Autodesk Fusion 360 part; units mm, degrees
(part 2 of 4)
sketch "top profile" plane through (0, 0, 1.6) normal (0, 0, 1) x (-1, 0, 0)
  circle A0 centre (-116.1773, 3.3688) radius 1.55
  line L0 (-280.938, -16.8245) -> (-266.937, -16.8245)
  line L1 (-266.937, -16.8245) -> (-266.937, -30.824)
  line L2 (-266.937, -30.824) -> (-280.938, -30.824)
  line L3 (-280.938, -30.824) -> (-280.938, -16.8245)
  line L4 (-197.772, -48.7839) -> (-183.986, -46.3532)
  line L5 (-183.986, -46.3532) -> (-181.555, -60.1405)
  line L6 (-181.555, -60.1405) -> (-195.341, -62.5711)
  line L7 (-195.341, -62.5711) -> (-197.772, -48.7839)
  line L8 (-176.582, -59.2624) -> (-179.013, -45.4752)
  line L9 (-179.013, -45.4752) -> (-165.224, -43.0445)
  line L10 (-165.224, -43.0445) -> (-162.793, -56.8318)
  line L11 (-162.793, -56.8318) -> (-176.582, -59.2624)
  line L12 (-45.4822, -49.874) -> (-59.4815, -49.874)
  line L13 (-59.4815, -49.874) -> (-59.4815, -35.8743)
  line L14 (-59.4815, -35.8743) -> (-45.4822, -35.8743)
  line L15 (-45.4822, -35.8743) -> (-45.4822, -49.874)
  line L16 (-176.444, -20.5521) -> (-190.233, -22.9829)
  line L17 (-190.233, -22.9829) -> (-192.664, -9.1956)
  line L18 (-192.664, -9.1957) -> (-178.876, -6.7634)
  line L19 (-178.876, -6.7634) -> (-176.444, -20.5521)
  line L20 (-281.226, -49.874) -> (-295.225, -49.874)
  line L21 (-295.225, -49.874) -> (-295.225, -35.8743)
  line L22 (-295.225, -35.8743) -> (-281.226, -35.8743)
  line L23 (-281.226, -35.8743) -> (-281.226, -49.874)
  line L24 (-109.921, -22.1561) -> (-123.708, -19.7253)
  line L25 (-123.708, -19.7253) -> (-121.277, -5.9366)
  line L26 (-121.277, -5.9366) -> (-107.49, -8.3688)
  line L27 (-107.49, -8.3688) -> (-109.921, -22.1561)
  line L28 (-349.994, -68.924) -> (-349.994, -54.9243)
  line L29 (-349.994, -54.9243) -> (-335.995, -54.9243)
  line L30 (-335.995, -54.9243) -> (-335.995, -68.924)
  line L31 (-335.995, -68.924) -> (-349.994, -68.924)
  line L32 (-257.125, -16.8245) -> (-243.126, -16.8245)
  line L33 (-243.126, -16.8245) -> (-243.126, -30.824)
  line L34 (-243.126, -30.824) -> (-257.125, -30.824)
  line L35 (-257.125, -30.824) -> (-257.125, -16.8245)
  line L36 (-12.1447, -73.9743) -> (-12.1447, -87.974)
  line L37 (-12.1447, -87.974) -> (-26.1441, -87.974)
  line L38 (-26.1441, -87.974) -> (-26.1441, -73.9743)
  line L39 (-26.1441, -73.9743) -> (-12.1447, -73.9743)
  line L40 (-193.416, -100.919) -> (-195.847, -87.1319)
  line L41 (-195.847, -87.1319) -> (-182.059, -84.7012)
  line L42 (-182.059, -84.7012) -> (-179.629, -98.4885)
  line L43 (-179.629, -98.4885) -> (-193.416, -100.919)
  line L44 (-177.086, -83.8232) -> (-163.299, -81.3925)
  line L45 (-163.299, -81.3925) -> (-160.868, -95.1812)
  line L46 (-160.868, -95.1812) -> (-174.655, -97.6119)
  line L47 (-174.655, -97.6119) -> (-177.086, -83.8232)
  line L48 (-189.775, -66.7177) -> (-175.988, -64.2867)
  line L49 (-175.988, -64.2867) -> (-173.557, -78.0743)
  line L50 (-173.557, -78.0743) -> (-187.343, -80.5049)
  line L51 (-187.343, -80.5049) -> (-189.775, -66.7177)
  line L52 (-200.82, -88.0085) -> (-198.389, -101.797)
  line L53 (-198.389, -101.797) -> (-212.176, -104.228)
  line L54 (-212.176, -104.228) -> (-214.607, -90.4392)
  line L55 (-214.607, -90.4392) -> (-200.82, -88.0085)
  line L56 (-117.5, -78.8515) -> (-131.287, -76.4205)
  line L57 (-131.287, -76.4205) -> (-128.856, -62.6332)
  line L58 (-128.856, -62.6332) -> (-115.069, -65.0642)
  line L59 (-115.069, -65.0642) -> (-117.5, -78.8515)
  line L60 (-111.428, -99.2657) -> (-125.214, -96.8347)
  line L61 (-125.214, -96.8347) -> (-122.783, -83.0474)
  line L62 (-122.783, -83.0474) -> (-108.996, -85.4784)
  line L63 (-108.996, -85.4784) -> (-111.428, -99.2657)
  circle A1 centre (-309.1199, -118.074) radius 1.55
  line L64 (-12.1447, -93.0243) -> (-12.1447, -107.024)
  line L65 (-12.1447, -107.024) -> (-26.1441, -107.024)
  line L66 (-26.1441, -107.024) -> (-26.1441, -93.0243)
  line L67 (-26.1441, -93.0243) -> (-12.1447, -93.0243)
  line L68 (-143.976, -93.5274) -> (-141.544, -79.7387)
  line L69 (-141.544, -79.7387) -> (-127.758, -82.1697)
  line L70 (-127.758, -82.1697) -> (-130.189, -95.9584)
  line L71 (-130.189, -95.9584) -> (-143.976, -93.5274)
  line L72 (-194.747, -67.5954) -> (-192.316, -81.3816)
  line L73 (-192.316, -81.3816) -> (-206.105, -83.8122)
  line L74 (-206.105, -83.8122) -> (-208.536, -70.0264)
  line L75 (-208.536, -70.0264) -> (-194.747, -67.5954)
  line L76 (-49.9565, -87.974) -> (-49.9565, -73.9743)
  line L77 (-49.9565, -73.9743) -> (-35.9572, -73.9743)
  line L78 (-35.9572, -73.9743) -> (-35.9572, -87.974)
  line L79 (-35.9572, -87.974) -> (-49.9565, -87.974)
  arc A2 (-176.1339, -7.7732) -> (-176.9451, -8.9317) centre (-175.9603, -8.758) ccw
  line L80 (-176.1339, -7.7732) -> (-170.6459, -6.8059)
  arc A3 (-169.4875, -7.6172) -> (-170.6459, -6.8059) centre (-170.4724, -7.7907) ccw
  line L81 (-169.4875, -7.6172) -> (-167.4915, -18.9424)
  arc A4 (-168.3027, -20.1008) -> (-167.4915, -18.9424) centre (-168.4764, -19.116) ccw
  line L82 (-168.3027, -20.1008) -> (-173.7893, -21.0686)
  arc A5 (-174.9478, -20.2574) -> (-173.7893, -21.0686) centre (-173.963, -20.0838) ccw
  line L83 (-174.9478, -20.2574) -> (-176.9451, -8.9317)
  line L84 (-255.032, -49.874) -> (-269.032, -49.874)
  line L85 (-269.032, -49.874) -> (-269.032, -35.8743)
  line L86 (-269.032, -35.8743) -> (-255.032, -35.8743)
  line L87 (-255.032, -35.8743) -> (-255.032, -49.874)
  line L88 (-98.9566, -12.3811) -> (-100.9548, -23.7064)
  arc A6 (-102.1133, -24.5174) -> (-100.9548, -23.7064) centre (-101.9395, -23.5327) ccw
  line L89 (-102.1133, -24.5174) -> (-107.6038, -23.5487)
  arc A7 (-108.4148, -22.3903) -> (-107.6038, -23.5487) centre (-107.43, -22.564) ccw
  line L90 (-108.4148, -22.3903) -> (-106.4177, -11.0651)
  arc A8 (-105.2592, -10.254) -> (-106.4177, -11.0651) centre (-105.4329, -11.2388) ccw
  line L91 (-105.2592, -10.254) -> (-99.7677, -11.2225)
  arc A9 (-98.9566, -12.3811) -> (-99.7677, -11.2225) centre (-99.9414, -12.2073) ccw
  line L92 (-132.669, -56.8318) -> (-130.238, -43.0445)
  line L93 (-130.238, -43.0445) -> (-116.451, -45.4752)
  line L94 (-116.451, -45.4752) -> (-118.882, -59.2624)
  line L95 (-118.882, -59.2624) -> (-132.669, -56.8318)
  line L96 (-249.982, -49.874) -> (-249.982, -35.8743)
  line L97 (-249.982, -35.8743) -> (-235.982, -35.8743)
  line L98 (-235.982, -35.8743) -> (-235.982, -49.874)
  line L99 (-235.982, -49.874) -> (-249.982, -49.874)
  line L100 (-106.193, -42.1569) -> (-119.98, -39.726)
  line L101 (-119.98, -39.726) -> (-117.549, -25.9388)
  line L102 (-117.549, -25.9388) -> (-103.762, -28.3697)
  line L103 (-103.762, -28.3697) -> (-106.193, -42.1569)
  line L104 (-28.5254, -35.8743) -> (-14.5259, -35.8743)
  line L105 (-14.5259, -35.8743) -> (-14.5259, -49.874)
  line L106 (-14.5259, -49.874) -> (-28.5254, -49.874)
  line L107 (-28.5254, -49.874) -> (-28.5254, -35.8743)
  line L108 (-136.31, -22.6315) -> (-122.524, -25.0624)
  line L109 (-122.524, -25.0624) -> (-124.955, -38.8482)
  line L110 (-124.955, -38.8482) -> (-138.741, -36.4173)
  line L111 (-138.741, -36.4173) -> (-136.31, -22.6315)
  line L112 (-283.556, -57.3947) -> (-283.556, -68.8941)
  arc A10 (-284.556, -69.8941) -> (-283.556, -68.8941) centre (-284.556, -68.8941) ccw
  line L113 (-284.556, -69.8941) -> (-290.13, -69.8941)
  arc A11 (-291.13, -68.8941) -> (-290.13, -69.8941) centre (-290.13, -68.8941) ccw
  line L114 (-291.13, -68.8941) -> (-291.13, -57.3947)
  arc A12 (-290.13, -56.3947) -> (-291.13, -57.3947) centre (-290.13, -57.3947) ccw
  line L115 (-290.13, -56.3947) -> (-284.556, -56.3947)
  arc A13 (-283.556, -57.3947) -> (-284.556, -56.3947) centre (-284.556, -57.3947) ccw
  line L116 (-98.7887, -29.2475) -> (-85.0015, -31.6784)
  line L117 (-85.0015, -31.6784) -> (-87.4339, -45.4642)
  line L118 (-87.4339, -45.4642) -> (-101.221, -43.0332)
  line L119 (-101.221, -43.0332) -> (-98.7887, -29.2475)
  line L120 (-326.182, -31.112) -> (-312.182, -31.112)
  line L121 (-312.182, -31.112) -> (-312.182, -45.1115)
  line L122 (-312.182, -45.1115) -> (-326.182, -45.1115)
  line L123 (-326.182, -45.1115) -> (-326.182, -31.112)
  line L124 (-28.812, -16.8245) -> (-28.812, -30.824)
  line L125 (-28.812, -30.824) -> (-42.8128, -30.824)
  line L126 (-42.8128, -30.824) -> (-42.8128, -16.8245)
  line L127 (-42.8128, -16.8245) -> (-28.812, -16.8245)
  line L128 (-312.182, -12.062) -> (-312.182, -26.0615)
  line L129 (-312.182, -26.0615) -> (-326.182, -26.0615)
  line L130 (-326.182, -26.0615) -> (-326.182, -12.062)
  line L131 (-326.182, -12.062) -> (-312.182, -12.062)
  line L132 (-225.494, -14.9848) -> (-211.708, -12.5525)
  line L133 (-211.708, -12.5525) -> (-209.276, -26.3412)
  line L134 (-209.276, -26.3412) -> (-223.063, -28.7721)
  line L135 (-223.063, -28.7721) -> (-225.494, -14.9848)
  line L136 (-331.232, -26.0615) -> (-345.232, -26.0615)
  line L137 (-345.232, -26.0615) -> (-345.232, -12.062)
  line L138 (-345.232, -12.062) -> (-331.232, -12.062)
  line L139 (-331.232, -12.062) -> (-331.232, -26.0615)
  line L140 (-175.482, -39.726) -> (-189.27, -42.1569)
  line L141 (-189.27, -42.1569) -> (-191.7, -28.3697)
  line L142 (-191.7, -28.3697) -> (-177.913, -25.9388)
  line L143 (-177.913, -25.9388) -> (-175.482, -39.726)
  line L144 (-82.459, -46.3419) -> (-80.0283, -32.5548)
  line L145 (-80.0283, -32.5548) -> (-66.2411, -34.9856)
  line L146 (-66.2411, -34.9856) -> (-68.6731, -48.7729)
  line L147 (-68.6731, -48.7729) -> (-82.459, -46.3419)
  line L148 (-196.674, -29.2475) -> (-194.243, -43.0332)
  line L149 (-194.243, -43.0332) -> (-208.03, -45.4642)
  line L150 (-208.03, -45.4642) -> (-210.461, -31.6784)
  line L151 (-210.461, -31.6784) -> (-196.674, -29.2475)
  line L152 (-5.0009, -16.8245) -> (-5.0009, -30.824)
  line L153 (-5.0009, -30.824) -> (-19.0004, -30.824)
  line L154 (-19.0004, -30.824) -> (-19.0004, -16.8245)
  line L155 (-19.0004, -16.8245) -> (-5.0009, -16.8245)
  line L156 (-311.47, -106.9941) -> (-311.47, -95.4943)
  arc A14 (-310.47, -94.4943) -> (-311.47, -95.4943) centre (-310.47, -95.4943) ccw
  line L157 (-310.47, -94.4943) -> (-304.895, -94.4943)
  arc A15 (-303.895, -95.4943) -> (-304.895, -94.4943) centre (-304.895, -95.4943) ccw
  line L158 (-303.895, -95.4943) -> (-303.895, -106.9941)
  arc A16 (-304.895, -107.9941) -> (-303.895, -106.9941) centre (-304.895, -106.9941) ccw
  line L159 (-304.895, -107.9941) -> (-310.47, -107.9941)
  arc A17 (-311.47, -106.9941) -> (-310.47, -107.9941) centre (-310.47, -106.9941) ccw
  arc A18 (-132.6638, -18.1157) -> (-131.8525, -19.274) centre (-131.679, -18.2892) ccw
  line L160 (-132.6638, -18.1157) -> (-130.6683, -6.7899)
  arc A19 (-129.5099, -5.9786) -> (-130.6683, -6.7899) centre (-129.6834, -6.9634) ccw
  line L161 (-129.5099, -5.9786) -> (-124.0183, -6.9465)
  arc A20 (-123.207, -8.1049) -> (-124.0183, -6.9465) centre (-124.1918, -7.9313) ccw
  line L162 (-123.207, -8.1049) -> (-125.2035, -19.4302)
  arc A21 (-126.3618, -20.2415) -> (-125.2035, -19.4302) centre (-126.1883, -19.2566) ccw
  line L163 (-126.3618, -20.2415) -> (-131.8525, -19.274)
  arc A22 (-37.6259, -49.8429) -> (-36.6259, -50.8429) centre (-36.6259, -49.8429) ccw
  line L164 (-37.6259, -49.8429) -> (-37.6259, -38.3436)
  arc A23 (-36.6259, -37.3436) -> (-37.6259, -38.3436) centre (-36.6259, -38.3436) ccw
  line L165 (-36.6259, -37.3436) -> (-31.0509, -37.3436)
  arc A24 (-30.0509, -38.3436) -> (-31.0509, -37.3436) centre (-31.0509, -38.3436) ccw
  line L166 (-30.0509, -38.3436) -> (-30.0509, -49.8429)
  arc A25 (-31.0509, -50.8429) -> (-30.0509, -49.8429) centre (-31.0509, -49.8429) ccw
  line L167 (-31.0509, -50.8429) -> (-36.6259, -50.8429)
  line L168 (-6.4253, -50.8429) -> (-12.0004, -50.8429)
  arc A26 (-13.0004, -49.8429) -> (-12.0004, -50.8429) centre (-12.0004, -49.8429) ccw
  line L169 (-13.0004, -49.8429) -> (-13.0004, -38.3436)
  arc A27 (-12.0004, -37.3436) -> (-13.0004, -38.3436) centre (-12.0004, -38.3436) ccw
  line L170 (-12.0004, -37.3436) -> (-6.4253, -37.3436)
  arc A28 (-5.4253, -38.3436) -> (-6.4253, -37.3436) centre (-6.4253, -38.3436) ccw
  line L171 (-5.4253, -38.3436) -> (-5.4253, -49.8429)
  arc A29 (-6.4253, -50.8429) -> (-5.4253, -49.8429) centre (-6.4253, -49.8429) ccw
  line L172 (-171.013, -63.4104) -> (-157.226, -60.9783)
  line L173 (-157.226, -60.9783) -> (-154.795, -74.7656)
  line L174 (-154.795, -74.7656) -> (-168.582, -77.1962)
  line L175 (-168.582, -77.1962) -> (-171.013, -63.4104)
  line L176 (-255.032, -73.9743) -> (-255.032, -87.974)
  line L177 (-255.032, -87.974) -> (-269.032, -87.974)
  line L178 (-269.032, -87.974) -> (-269.032, -73.9743)
  line L179 (-269.032, -73.9743) -> (-255.032, -73.9743)
  line L180 (-306.655, -54.9243) -> (-292.655, -54.9243)
  line L181 (-292.655, -54.9243) -> (-292.655, -68.924)
  line L182 (-292.655, -68.924) -> (-306.655, -68.924)
  line L183 (-306.655, -68.924) -> (-306.655, -54.9243)
  line L184 (-60.1694, -55.3999) -> (-62.6001, -69.1871)
  line L185 (-62.6001, -69.1871) -> (-76.3873, -66.7561)
  line L186 (-76.3873, -66.7561) -> (-73.9567, -52.9689)
  line L187 (-73.9567, -52.9689) -> (-60.1694, -55.3999)
  line L188 (-311.894, -73.9743) -> (-297.895, -73.9743)
  line L189 (-297.895, -73.9743) -> (-297.895, -87.974)
  line L190 (-297.895, -87.974) -> (-311.894, -87.974)
  line L191 (-311.894, -87.974) -> (-311.894, -73.9743)
  line L192 (-345.232, -73.9743) -> (-331.232, -73.9743)
  line L193 (-331.232, -73.9743) -> (-331.232, -87.974)
  line L194 (-331.232, -87.974) -> (-345.232, -87.974)
  line L195 (-345.232, -87.974) -> (-345.232, -73.9743)
  line L196 (-86.1882, -26.3412) -> (-83.7558, -12.5525)
  line L197 (-83.7558, -12.5525) -> (-69.9685, -14.9848)
  line L198 (-69.9685, -14.9848) -> (-72.3995, -28.7721)
  line L199 (-72.3995, -28.7721) -> (-86.1882, -26.3412)
  line L200 (-170.509, -38.8482) -> (-172.94, -25.0624)
  line L201 (-172.94, -25.0624) -> (-159.153, -22.6315)
  line L202 (-159.153, -22.6315) -> (-156.722, -36.4173)
  line L203 (-156.722, -36.4173) -> (-170.509, -38.8482)
  line L204 (-215.434, -32.5548) -> (-213.003, -46.3419)
  line L205 (-213.003, -46.3419) -> (-226.791, -48.7729)
  line L206 (-226.791, -48.7729) -> (-229.222, -34.9856)
  line L207 (-229.222, -34.9856) -> (-215.434, -32.5548)
  arc A30 (-199.1959, -24.5335) -> (-198.0375, -25.3445) centre (-198.2111, -24.3597) ccw
  line L208 (-199.1959, -24.5335) -> (-201.1942, -13.2086)
  arc A31 (-200.3832, -12.0501) -> (-201.1942, -13.2086) centre (-200.2094, -13.0348) ccw
  line L209 (-200.3832, -12.0501) -> (-194.8954, -11.0818)
  arc A32 (-193.7369, -11.8929) -> (-194.8954, -11.0818) centre (-194.7217, -12.0666) ccw
  line L210 (-193.7369, -11.8929) -> (-191.7396, -23.2186)
  arc A33 (-192.5507, -24.3771) -> (-191.7396, -23.2186) centre (-192.7244, -23.3923) ccw
  line L211 (-192.5507, -24.3771) -> (-198.0375, -25.3445)
  line L212 (-275.7, -54.9243) -> (-261.699, -54.9243)
  line L213 (-261.699, -54.9243) -> (-261.699, -68.924)
  line L214 (-261.699, -68.924) -> (-275.7, -68.924)
  line L215 (-275.7, -68.924) -> (-275.7, -54.9243)
  line L216 (-242.649, -54.9243) -> (-242.649, -68.924)
  line L217 (-242.649, -68.924) -> (-256.65, -68.924)
  line L218 (-256.65, -68.924) -> (-256.65, -54.9243)
  line L219 (-256.65, -54.9243) -> (-242.649, -54.9243)
  line L220 (-75.0051, -86.3438) -> (-72.5745, -72.5565)
  line L221 (-72.5745, -72.5565) -> (-58.7872, -74.9886)
  line L222 (-58.7872, -74.9886) -> (-61.2179, -88.7748)
  line L223 (-61.2179, -88.7748) -> (-75.0051, -86.3438)
  line L224 (-214.103, -65.8784) -> (-216.534, -52.0912)
  line L225 (-216.534, -52.0912) -> (-202.747, -49.6605)
  line L226 (-202.747, -49.6605) -> (-200.314, -63.4478)
  line L227 (-200.314, -63.4478) -> (-214.103, -65.8784)
  line L228 (-38.8137, -54.9243) -> (-38.8137, -68.924)
  line L229 (-38.8137, -68.924) -> (-52.8147, -68.924)
  line L230 (-52.8147, -68.924) -> (-52.8147, -54.9243)
  line L231 (-52.8147, -54.9243) -> (-38.8137, -54.9243)
  line L232 (-111.478, -46.3532) -> (-97.6905, -48.7839)
  line L233 (-97.6905, -48.7839) -> (-100.122, -62.5711)
  line L234 (-100.122, -62.5711) -> (-113.909, -60.1405)
  line L235 (-113.909, -60.1405) -> (-111.478, -46.3532)
  line L236 (-96.3083, -68.3715) -> (-98.7393, -82.1588)
  line L237 (-98.7393, -82.1588) -> (-112.527, -79.7278)
  line L238 (-112.527, -79.7278) -> (-110.096, -65.9405)
  line L239 (-110.096, -65.9405) -> (-96.3083, -68.3715)
  line L240 (-219.581, -91.3172) -> (-217.15, -105.104)
  line L241 (-217.15, -105.104) -> (-230.937, -107.535)
  line L242 (-230.937, -107.535) -> (-233.368, -93.7479)
  line L243 (-233.368, -93.7479) -> (-219.581, -91.3172)
  line L244 (-90.2353, -88.7857) -> (-92.6663, -102.574)
  line L245 (-92.6663, -102.574) -> (-106.455, -100.143)
  line L246 (-106.455, -100.143) -> (-104.024, -86.3547)
  line L247 (-104.024, -86.3547) -> (-90.2353, -88.7857)
  line L248 (-274.082, -87.974) -> (-288.082, -87.974)
  line L249 (-288.082, -87.974) -> (-288.082, -73.9743)
  line L250 (-288.082, -73.9743) -> (-274.082, -73.9743)
  line L251 (-274.082, -73.9743) -> (-274.082, -87.974)
  line L252 (-211.077, -84.6899) -> (-224.864, -87.1209)
  line L253 (-224.864, -87.1209) -> (-227.295, -73.3337)
  line L254 (-227.295, -73.3337) -> (-213.509, -70.9027)
  line L255 (-213.509, -70.9027) -> (-211.077, -84.6899)
  circle A34 centre (-133.6233, -118.074) radius 1.55
  line L256 (-219.075, -66.7561) -> (-232.862, -69.1871)
  line L257 (-232.862, -69.1871) -> (-235.293, -55.3999)
  line L258 (-235.293, -55.3999) -> (-221.506, -52.9689)
  line L259 (-221.506, -52.9689) -> (-219.075, -66.7561)
  line L260 (-288.37, -107.024) -> (-302.369, -107.024)
  line L261 (-302.369, -107.024) -> (-302.369, -93.0243)
  line L262 (-302.369, -93.0243) -> (-288.37, -93.0243)
  line L263 (-288.37, -93.0243) -> (-288.37, -107.024)
  line L264 (-87.6928, -103.451) -> (-85.2622, -89.6634)
  line L265 (-85.2622, -89.6634) -> (-71.476, -92.0944)
  line L266 (-71.476, -92.0944) -> (-73.9069, -105.882)
  line L267 (-73.9069, -105.882) -> (-87.6928, -103.451)
  line L268 (-93.7659, -83.0365) -> (-91.3349, -69.2492)
  line L269 (-91.3349, -69.2492) -> (-77.5476, -71.6802)
  line L270 (-77.5476, -71.6802) -> (-79.9786, -85.4675)
  line L271 (-79.9786, -85.4675) -> (-93.7659, -83.0365)
  line L272 (-249.982, -73.9743) -> (-235.982, -73.9743)
  line L273 (-235.982, -73.9743) -> (-235.982, -87.974)
  line L274 (-235.982, -87.974) -> (-249.982, -87.974)
  line L275 (-249.982, -87.974) -> (-249.982, -73.9743)
  line L276 (-285.844, -94.4943) -> (-280.269, -94.4943)
  arc A35 (-279.269, -95.4943) -> (-280.269, -94.4943) centre (-280.269, -95.4943) ccw
  line L277 (-279.269, -95.4943) -> (-279.269, -106.9941)
  arc A36 (-280.269, -107.9941) -> (-279.269, -106.9941) centre (-280.269, -106.9941) ccw
  line L278 (-280.269, -107.9941) -> (-285.844, -107.9941)
  arc A37 (-286.844, -106.9941) -> (-285.844, -107.9941) centre (-285.844, -106.9941) ccw
  line L279 (-286.844, -106.9941) -> (-286.844, -95.4943)
  arc A38 (-285.844, -94.4943) -> (-286.844, -95.4943) centre (-285.844, -95.4943) ccw
  line L280 (-254.744, -93.0243) -> (-240.745, -93.0243)
  line L281 (-240.745, -93.0243) -> (-240.745, -107.024)
  line L282 (-240.745, -107.024) -> (-254.744, -107.024)
  line L283 (-254.744, -107.024) -> (-254.744, -93.0243)
  circle A39 centre (-221.3716, -118.074) radius 1.55
  line L284 (-259.795, -107.024) -> (-273.794, -107.024)
  line L285 (-273.794, -107.024) -> (-273.794, -93.0243)
  line L286 (-273.794, -93.0243) -> (-259.795, -93.0243)
  line L287 (-259.795, -93.0243) -> (-259.795, -107.024)
  circle A40 centre (-281.3904, -1.95) radius 1.55
  arc A41 (-315.754, -68.8941) -> (-314.754, -69.8941) centre (-314.754, -68.8941) ccw
  line L288 (-315.754, -68.8941) -> (-315.754, -57.3947)
  arc A42 (-314.754, -56.3947) -> (-315.754, -57.3947) centre (-314.754, -57.3947) ccw
  line L289 (-314.754, -56.3947) -> (-309.18, -56.3947)
  arc A43 (-308.18, -57.3947) -> (-309.18, -56.3947) centre (-309.18, -57.3947) ccw
  line L290 (-308.18, -57.3947) -> (-308.18, -68.8941)
  arc A44 (-309.18, -69.8941) -> (-308.18, -68.8941) centre (-309.18, -68.8941) ccw
  line L291 (-309.18, -69.8941) -> (-314.754, -69.8941)
  circle A45 centre (-179.2893, 3.3688) radius 1.55
  line L292 (-31.1947, -93.0243) -> (-31.1947, -107.024)
  line L293 (-31.1947, -107.024) -> (-45.194, -107.024)
  line L294 (-45.194, -107.024) -> (-45.194, -93.0243)
  line L295 (-45.194, -93.0243) -> (-31.1947, -93.0243)
  line L296 (-307.132, -12.062) -> (-293.132, -12.062)
  line L297 (-293.132, -12.062) -> (-293.132, -26.0615)
  line L298 (-293.132, -26.0615) -> (-307.132, -26.0615)
  line L299 (-307.132, -26.0615) -> (-307.132, -12.062)
  line L300 (-7.8576, -68.924) -> (-26.6209, -68.924)
  line L301 (-26.6209, -68.924) -> (-26.6209, -54.9243)
  line L302 (-26.6209, -54.9243) -> (-7.8576, -54.9243)
  line L303 (-55.1448, -109.19) -> (-68.9335, -106.759)
  line L304 (-68.9335, -106.759) -> (-66.5014, -92.9707)
  line L305 (-66.5014, -92.9707) -> (-52.7142, -95.4017)
  line L306 (-52.7142, -95.4017) -> (-55.1448, -109.19)
  circle A46 centre (-45.875, -118.074) radius 1.55
  line L307 (-95.148, -63.4478) -> (-92.7171, -49.6605)
  line L308 (-92.7171, -49.6605) -> (-78.9298, -52.0912)
  line L309 (-78.9298, -52.0912) -> (-81.3608, -65.8784)
  line L310 (-81.3608, -65.8784) -> (-95.148, -63.4478)
  circle A47 centre (-43.8415, -1.95) radius 1.55
  line L311 (-326.47, -107.024) -> (-340.469, -107.024)
  line L312 (-340.469, -107.024) -> (-340.469, -93.0243)
  line L313 (-340.469, -93.0243) -> (-326.47, -93.0243)
  line L314 (-326.47, -93.0243) -> (-326.47, -107.024)
  arc A48 (-40.125, -115.524) -> (-42.375, -117.774) centre (-40.125, -117.774) ccw
  line L315 (-40.125, -115.524) -> (-2.0009, -115.524)
  arc A49 (-2.0009, -115.524) -> (3.4991, -110.024) centre (-2.0009, -110.024) ccw
  line L316 (3.4991, -110.024) -> (3.4991, -10)
  arc A50 (3.4991, -10) -> (-2.0009, -4.5) centre (-2.0009, -10) ccw
  line L317 (-2.0009, -4.5) -> (-38.0915, -4.5)
  arc A51 (-40.3415, -2.25) -> (-38.0915, -4.5) centre (-38.0915, -2.25) ccw
  line L318 (-40.3415, -2.25) -> (-40.3415, -1.7)
  arc A52 (-40.3415, -1.7) -> (-43.5915, 1.55) centre (-43.5915, -1.7) ccw
  line L319 (-43.5915, 1.55) -> (-44.0915, 1.55)
  arc A53 (-44.0915, 1.55) -> (-47.3415, -1.7) centre (-44.0915, -1.7) ccw
  line L320 (-47.3415, -1.7) -> (-47.3415, -2.25)
  arc A54 (-49.5915, -4.5) -> (-47.3415, -2.25) centre (-49.5915, -2.25) ccw
  line L321 (-49.5915, -4.5) -> (-85.6822, -4.5)
  arc A55 (-86.8114, -4.4012) -> (-85.6822, -4.5) centre (-85.6822, 2) ccw
  line L322 (-86.8114, -4.4012) -> (-110.9577, -0.1414)
  arc A56 (-112.7826, 2.4653) -> (-110.9577, -0.1414) centre (-110.5668, 2.0744) ccw
  line L323 (-112.7826, 2.4653) -> (-112.687, 3.007)
  arc A57 (-112.687, 3.007) -> (-115.323, 6.7722) centre (-115.8876, 3.5716) ccw
  line L324 (-115.323, 6.7722) -> (-115.8154, 6.859)
  arc A58 (-115.8154, 6.859) -> (-119.5806, 4.2231) centre (-116.38, 3.6585) ccw
  line L325 (-119.5806, 4.2231) -> (-119.6762, 3.6815)
  arc A59 (-122.2828, 1.8566) -> (-119.6762, 3.6815) centre (-121.8919, 4.0724) ccw
  line L326 (-122.2828, 1.8566) -> (-146.4291, 6.1164)
  arc A60 (-146.4291, 6.1164) -> (-149.035, 6.1164) centre (-147.7321, -1.2696) ccw
  line L327 (-149.035, 6.1164) -> (-173.1838, 1.8565)
  arc A61 (-175.7904, 3.6814) -> (-173.1838, 1.8565) centre (-173.5747, 4.0723) ccw
  line L328 (-175.7904, 3.6814) -> (-175.886, 4.2231)
  arc A62 (-175.886, 4.2231) -> (-179.6512, 6.859) centre (-179.0866, 3.6585) ccw
  line L329 (-179.6512, 6.859) -> (-180.1436, 6.7722)
  arc A63 (-180.1436, 6.7722) -> (-182.7796, 3.007) centre (-179.579, 3.5716) ccw
  line L330 (-182.7796, 3.007) -> (-182.684, 2.4654)
  arc A64 (-184.5089, -0.1413) -> (-182.684, 2.4654) centre (-184.8998, 2.0745) ccw
  line L331 (-184.5089, -0.1413) -> (-208.6577, -4.4012)
  arc A65 (-209.7869, -4.5) -> (-208.6577, -4.4012) centre (-209.7869, 2) ccw
  line L332 (-209.7869, -4.5) -> (-275.6404, -4.5)
  arc A66 (-277.8904, -2.25) -> (-275.6404, -4.5) centre (-275.6404, -2.25) ccw
  line L333 (-277.8904, -2.25) -> (-277.8904, -1.7)
  arc A67 (-277.8904, -1.7) -> (-281.1404, 1.55) centre (-281.1404, -1.7) ccw
  line L334 (-281.1404, 1.55) -> (-281.6404, 1.55)
  arc A68 (-281.6404, 1.55) -> (-284.8904, -1.7) centre (-281.6404, -1.7) ccw
  line L335 (-284.8904, -1.7) -> (-284.8904, -2.25)
  arc A69 (-287.1404, -4.5) -> (-284.8904, -2.25) centre (-287.1404, -2.25) ccw
  line L336 (-287.1404, -4.5) -> (-352.994, -4.5)
  arc A70 (-352.994, -4.5) -> (-358.494, -10) centre (-352.994, -10) ccw
  line L337 (-358.494, -10) -> (-358.494, -110.024)
  arc A71 (-358.494, -110.024) -> (-352.994, -115.524) centre (-352.994, -110.024) ccw
  line L338 (-352.994, -115.524) -> (-314.8699, -115.524)
  arc A72 (-312.6199, -117.774) -> (-314.8699, -115.524) centre (-314.8699, -117.774) ccw
  line L339 (-312.6199, -117.774) -> (-312.6199, -118.324)
  arc A73 (-312.6199, -118.324) -> (-309.3699, -121.574) centre (-309.3699, -118.324) ccw
  line L340 (-309.3699, -121.574) -> (-308.8699, -121.574)
  arc A74 (-308.8699, -121.574) -> (-305.6199, -118.324) centre (-308.8699, -118.324) ccw
  line L341 (-305.6199, -118.324) -> (-305.6199, -117.774)
  arc A75 (-303.3699, -115.524) -> (-305.6199, -117.774) centre (-303.3699, -117.774) ccw
  line L342 (-303.3699, -115.524) -> (-227.1216, -115.524)
  arc A76 (-224.8716, -117.774) -> (-227.1216, -115.524) centre (-227.1216, -117.774) ccw
  line L343 (-224.8716, -117.774) -> (-224.8716, -118.324)
  arc A77 (-224.8716, -118.324) -> (-221.6216, -121.574) centre (-221.6216, -118.324) ccw
  line L344 (-221.6216, -121.574) -> (-221.1216, -121.574)
  arc A78 (-221.1216, -121.574) -> (-217.8716, -118.324) centre (-221.1216, -118.324) ccw
  line L345 (-217.8716, -118.324) -> (-217.8716, -117.774)
  arc A79 (-215.6216, -115.524) -> (-217.8716, -117.774) centre (-215.6216, -117.774) ccw
  line L346 (-215.6216, -115.524) -> (-139.3733, -115.524)
  arc A80 (-137.1233, -117.774) -> (-139.3733, -115.524) centre (-139.3733, -117.774) ccw
  line L347 (-137.1233, -117.774) -> (-137.1233, -118.324)
  arc A81 (-137.1233, -118.324) -> (-133.8733, -121.574) centre (-133.8733, -118.324) ccw
  line L348 (-133.8733, -121.574) -> (-133.3733, -121.574)
  arc A82 (-133.3733, -121.574) -> (-130.1233, -118.324) centre (-133.3733, -118.324) ccw
  line L349 (-130.1233, -118.324) -> (-130.1233, -117.774)
  arc A83 (-127.8733, -115.524) -> (-130.1233, -117.774) centre (-127.8733, -117.774) ccw
  line L350 (-127.8733, -115.524) -> (-51.625, -115.524)
  arc A84 (-49.375, -117.774) -> (-51.625, -115.524) centre (-51.625, -117.774) ccw
  line L351 (-49.375, -117.774) -> (-49.375, -118.324)
  arc A85 (-49.375, -118.324) -> (-46.125, -121.574) centre (-46.125, -118.324) ccw
  line L352 (-46.125, -121.574) -> (-45.625, -121.574)
  arc A86 (-45.625, -121.574) -> (-42.375, -118.324) centre (-45.625, -118.324) ccw
  line L353 (-42.375, -118.324) -> (-42.375, -117.774)
  line L354 (-9.6197, -90.5036) -> (-9.6197, -109.6269)
  line L355 (-124.833, -80.1215) -> (-124.8331, -80.1224)
  line L356 (-146.7974, -95.4313) -> (-143.5473, -76.8223)
  line L357 (-161.2642, -78.4117) -> (-157.9507, -97.2461)
  line L358 (-314.419, -109.5323) -> (-314.419, -90.5497)
  line L359 (-319.1815, -90.5517) -> (-319.1815, -71.5041)
  line L360 (-321.0862, -71.5048) -> (-321.0862, -52.461)
  line L361 (-304.8937, -52.4518) -> (-304.8937, -33.4289)
  line L362 (-285.8442, -33.4146) -> (-285.8442, -14.2995)
  line L363 (-309.6529, -28.5419) -> (-309.6278, -47.5612)
  line L364 (-309.6278, -47.5612) -> (-328.7886, -47.5463)
  line L365 (-328.7886, -47.5463) -> (-328.7195, -28.5938)
  line L366 (-290.6022, -9.5322) -> (-290.6316, -28.5492)
  line L367 (-347.758, -28.5945) -> (-347.7568, -9.5286)
  line L368 (-238.2191, -14.2995) -> (-238.2191, -33.3824)
  line L369 (-165.2794, -1.8104) -> (-161.9715, -20.5648)
  line L370 (-142.7976, -18.9304) -> (-139.4916, -0.1632)
  line L371 (-2.9429, -52.4065) -> (-2.9285, -71.4484)
  line L372 (-4.8442, -71.4454) -> (-4.83, -90.5)
  line L373 (-134.3065, -78.4527) -> (-130.9677, -59.7792)
  line L374 (-135.6283, -58.9666) -> (-132.2992, -40.1468)
  line L375 (-141.7263, -38.4919) -> (-138.3753, -19.7094)
  line L376 (-157.1048, -19.7064) -> (-153.8077, -38.4041)
  line L377 (-163.1887, -40.0463) -> (-159.882, -58.7999)
  line L378 (-155.1908, -57.9794) -> (-151.8783, -76.7664)
  line L379 (-290.6316, -28.5492) -> (-309.6529, -28.5419)
  line L380 (-328.7195, -28.5938) -> (-347.758, -28.5945)
  line L381 (-290.6022, -9.5322) -> (-347.7568, -9.5286)
  line L382 (-82.0765, -29.6297) -> (-68.0398, -32.1045)
  line L383 (-151.8783, -76.7664) -> (-161.2642, -78.4117)
  line L384 (-155.1908, -57.9794) -> (-159.882, -58.7999)
  line L385 (-153.8077, -38.4041) -> (-163.1887, -40.0463)
  line L386 (-157.1048, -19.7064) -> (-161.9715, -20.5648)
  line L387 (-138.3753, -19.7094) -> (-142.7976, -18.9304)
  line L388 (-132.2992, -40.1468) -> (-141.7263, -38.4919)
  line L389 (-130.9677, -59.7792) -> (-135.6283, -58.9666)
  line L390 (-134.3065, -78.4527) -> (-143.5473, -76.8223)
  line L391 (-4.83, -90.5) -> (-9.6197, -90.5036)
  line L392 (-2.9285, -71.4484) -> (-4.8442, -71.4454)
  line L393 (-0.2449, -52.396) -> (-2.9429, -52.4065)
  line L394 (-0.0552, -14.3048) -> (-47.7152, -14.289)
  line L395 (-0.2449, -52.396) -> (-0.0552, -14.3048)
  line L396 (-64.7322, -13.3439) -> (-139.4916, -0.1632)
  line L397 (-64.7322, -13.3439) -> (-68.0398, -32.1045)
  line L398 (-165.2794, -1.8104) -> (-230.7205, -13.3717)
  line L399 (-230.7205, -13.3717) -> (-227.4154, -32.1328)
  line L400 (-238.2191, -14.2995) -> (-285.8442, -14.2995)
  line L401 (-285.8442, -33.4146) -> (-304.8937, -33.4289)
  line L402 (-304.8937, -52.4518) -> (-321.0862, -52.461)
  line L403 (-319.1815, -71.5041) -> (-321.0862, -71.5048)
  line L404 (-314.419, -90.5497) -> (-319.1815, -90.5517)
  line L405 (-47.7152, -14.289) -> (-47.7616, -33.3369)
  arc A87 (-68.0398, -32.1045) -> (-47.7616, -33.3369) centre (-46.6903, 151.7378) ccw
  arc A88 (-238.2191, -33.3824) -> (-227.4154, -32.1328) centre (-243.2466, 57.4136) ccw
  line L406 (-7.8576, -54.9243) -> (-7.8576, -68.924)
  line L407 (3.4991, -110.024) -> (3.4991, -10)
  arc A89 (-2.0009, -115.524) -> (3.4991, -110.024) centre (-2.0009, -110.024) ccw
  arc A90 (3.4991, -10) -> (-2.0009, -4.5) centre (-2.0009, -10) ccw
  arc A91 (-86.8114, -4.4012) -> (-85.6822, -4.5) centre (-85.6822, 2) ccw
  arc A92 (-146.4291, 6.1164) -> (-149.035, 6.1164) centre (-147.7321, -1.2696) ccw
  arc A93 (-209.7869, -4.5) -> (-208.6577, -4.4012) centre (-209.7869, 2) ccw
  line L408 (-184.5089, -0.1413) -> (-208.6577, -4.4012)
  line L409 (-86.8114, -4.4012) -> (-110.9577, -0.1414)
  arc A94 (-352.994, -4.5) -> (-358.494, -10) centre (-352.994, -10) ccw
  line L410 (-358.494, -10) -> (-358.494, -110.024)
  arc A95 (-358.494, -110.024) -> (-352.994, -115.524) centre (-352.994, -110.024) ccw
  line L411 (-352.994, -115.524) -> (-2.0009, -115.524)
  line L412 (-2.0009, -4.5) -> (-85.6822, -4.5)
  line L413 (-110.9577, -0.1414) -> (-146.4291, 6.1164)
  line L414 (-149.035, 6.1164) -> (-184.5089, -0.1413)
  line L415 (-209.7869, -4.5) -> (-352.994, -4.5)
  line L416 (-352.994, -124.024) -> (-2.0009, -124.024)
  arc A96 (-2.0009, -124.024) -> (11.9991, -110.024) centre (-2.0009, -110.024) ccw
  line L417 (11.9991, -110.024) -> (11.9991, -10)
  arc A97 (11.9991, -10) -> (-2.0009, 4) centre (-2.0009, -10) ccw
  line L418 (-2.0009, 4) -> (-85.5071, 4)
  line L419 (-85.5071, 4) -> (-109.481, 8.2294)
  line L420 (-109.481, 8.2294) -> (-144.9524, 14.4871)
  arc A98 (-144.9524, 14.4871) -> (-150.5116, 14.4871) centre (-147.7321, -1.2696) ccw
  line L421 (-150.5116, 14.4871) -> (-185.9855, 8.2295)
  line L422 (-185.9855, 8.2295) -> (-209.9619, 4)
  line L423 (-209.9619, 4) -> (-352.994, 4)
  arc A99 (-352.994, 4) -> (-366.994, -10) centre (-352.994, -10) ccw
  line L424 (-366.994, -10) -> (-366.994, -110.024)
  arc A100 (-366.994, -110.024) -> (-352.994, -124.024) centre (-352.994, -110.024) ccw
  line L425 (-326.47, -107.024) -> (-340.469, -93.0243) construction
  line L426 (-340.469, -107.024) -> (-326.47, -93.0243) construction
  line L427 (-331.232, -87.974) -> (-345.232, -73.9743) construction
  line L428 (-331.232, -73.9743) -> (-345.232, -87.974) construction
  line L429 (-335.995, -68.924) -> (-349.994, -54.9243) construction
  line L430 (-335.995, -54.9243) -> (-349.994, -68.924) construction
  circle A101 centre (-342.9945, -61.9242) radius 4.125
  circle A102 centre (-338.232, -80.9741) radius 4.125
  circle A103 centre (-333.4695, -100.0241) radius 4.125
  line L431 (-9.6197, -109.6269) -> (-47.719, -109.549)
  line L432 (-53.0965, -112.1151) -> (-146.7974, -95.4313)
  line L433 (-53.0965, -112.1151) -> (-47.719, -109.549)
  line L434 (-157.9507, -97.2461) -> (-232.9852, -110.4601)
  line L435 (-232.9852, -110.4601) -> (-238.22, -109.549)
  line L436 (-238.22, -109.549) -> (-314.419, -109.5323)
  line L437 (-314.919, -108.3659) -> (-314.919, -91.0499)
  line L438 (-314.919, -91.0499) -> (-318.0141, -91.0512)
  line L439 (-319.6815, -89.3845) -> (-319.6815, -72.0042)
  line L440 (-319.6815, -72.0042) -> (-319.919, -72.0043)
  line L441 (-321.5862, -70.3377) -> (-321.5862, -53.627)
  line L442 (-305.3937, -51.9521) -> (-319.9205, -51.9603)
  line L443 (-305.3937, -51.9521) -> (-305.3937, -34.5947)
  line L444 (-286.3442, -32.9149) -> (-303.7283, -32.928)
  line L445 (-286.3442, -32.9149) -> (-286.3442, -15.4662)
  line L446 (-239.3858, -13.7995) -> (-284.6776, -13.7995)
  line L447 (-237.7191, -15.4662) -> (-237.7191, -31.0628)
  arc A104 (-235.9174, -32.724) -> (-229.6794, -31.998) centre (-243.2466, 57.4136) ccw
  line L448 (-231.0106, -14.6069) -> (-228.2881, -30.061)
  line L449 (-166.5156, -1.521) -> (-229.6592, -12.6764)
  line L450 (-164.5843, -2.8728) -> (-161.566, -19.9855)
  line L451 (-158.3407, -19.4167) -> (-161.566, -19.9855)
  line L452 (-156.4098, -20.7686) -> (-153.5181, -37.1669)
  line L453 (-154.8721, -39.098) -> (-162.6093, -40.4525)
  line L454 (-162.6093, -40.4525) -> (-159.4763, -58.2214)
  line L455 (-156.4246, -57.6876) -> (-159.4763, -58.2214)
  line L456 (-154.4961, -59.04) -> (-151.5886, -75.5295)
  line L457 (-152.9422, -77.4605) -> (-160.6851, -78.8178)
  line L458 (-160.6851, -78.8178) -> (-157.6604, -96.0106)
  line L459 (-159.0128, -97.9408) -> (-232.6973, -110.9171)
  line L460 (-233.2721, -110.9177) -> (-238.1216, -110.0736)
  line L461 (-238.407, -110.049) -> (-313.2527, -110.0326)
  line L462 (-348.2579, -27.4277) -> (-348.2569, -10.6952)
  line L463 (-291.7706, -9.0321) -> (-346.5901, -9.0287)
  line L464 (-290.104, -10.7013) -> (-290.1298, -27.3847)
  line L465 (-291.7971, -29.0488) -> (-309.1522, -29.0421)
  line L466 (-309.1522, -29.0421) -> (-309.1294, -46.3914)
  line L467 (-310.7973, -48.0603) -> (-327.619, -48.0472)
  line L468 (-329.2843, -46.3744) -> (-329.2213, -29.0938)
  line L469 (-329.2213, -29.0938) -> (-346.5912, -29.0945)
  arc A105 (-65.6759, -31.861) -> (-49.9524, -32.8112) centre (-46.6903, 151.7378) ccw
  line L470 (-48.218, -15.452) -> (-48.2563, -31.1489)
  line L471 (-1.2271, -13.8044) -> (-46.5508, -13.7894)
  line L472 (0.2609, -51.2421) -> (0.439, -15.4793)
  line L473 (-1.3993, -52.9005) -> (-2.4426, -52.9046)
  line L474 (-2.4426, -52.9046) -> (-2.4294, -70.2787)
  line L475 (-4.0987, -71.9466) -> (-4.3438, -71.9462)
  line L476 (-4.3438, -71.9462) -> (-4.3309, -89.333)
  line L477 (-5.9963, -91.0009) -> (-9.1197, -91.0032)
  line L478 (-9.1197, -91.0032) -> (-9.1197, -108.4579)
  line L479 (-10.7898, -110.1245) -> (-47.2272, -110.05)
  line L480 (-52.543, -112.405) -> (-47.9484, -110.2125)
  line L481 (-53.553, -112.5417) -> (-145.7402, -96.1274)
  line L482 (-147.0899, -94.1998) -> (-144.2409, -77.8876)
  line L483 (-134.7109, -77.8736) -> (-142.3095, -76.533)
  line L484 (-134.7109, -77.8736) -> (-131.5483, -60.1855)
  line L485 (-131.5483, -60.1855) -> (-134.562, -59.6601)
  line L486 (-135.9169, -57.7279) -> (-132.8787, -40.5527)
  line L487 (-132.8787, -40.5527) -> (-140.6605, -39.1866)
  line L488 (-142.0131, -37.2523) -> (-138.9556, -20.1149)
  line L489 (-138.9556, -20.1149) -> (-141.7354, -19.6252)
  line L490 (-143.0876, -17.6947) -> (-140.1864, -1.2256)
  line L491 (-65.7943, -12.6489) -> (-138.2556, 0.1266)
  line L492 (-64.4423, -14.5796) -> (-67.1459, -29.9138)
  arc A106 (-46.5508, -13.7894) -> (-48.218, -15.452) centre (-46.5514, -15.4561) ccw
  arc A107 (-49.9524, -32.8112) -> (-48.2563, -31.1489) centre (-49.923, -31.1448) ccw
  arc A108 (-67.1459, -29.9138) -> (-65.6759, -31.861) centre (-65.5045, -30.2032) ccw
  arc A109 (-64.4423, -14.5796) -> (-65.7943, -12.6489) centre (-66.0837, -14.2903) ccw
  arc A110 (0.439, -15.4793) -> (-1.2271, -13.8044) centre (-1.2277, -15.471) ccw
  arc A111 (-1.3993, -52.9005) -> (0.2609, -51.2421) centre (-1.4058, -51.2338) ccw
  arc A112 (-4.0987, -71.9466) -> (-2.4294, -70.2787) centre (-4.0961, -70.28) ccw
  arc A113 (-5.9963, -91.0009) -> (-4.3309, -89.333) centre (-5.9976, -89.3342) ccw
  arc A114 (-10.7898, -110.1245) -> (-9.1197, -108.4579) centre (-10.7864, -108.4579) ccw
  arc A115 (-47.2272, -110.05) -> (-47.9484, -110.2125) centre (-47.2306, -111.7167) ccw
  arc A116 (-53.553, -112.5417) -> (-52.543, -112.405) centre (-53.2608, -110.9008) ccw
  arc A117 (-147.0899, -94.1998) -> (-145.7402, -96.1274) centre (-145.448, -94.4865) ccw
  arc A118 (-142.3095, -76.533) -> (-144.2409, -77.8876) centre (-142.5991, -78.1743) ccw
  arc A119 (-135.9169, -57.7279) -> (-134.562, -59.6601) centre (-134.2757, -58.0182) ccw
  arc A120 (-142.0131, -37.2523) -> (-140.6605, -39.1866) centre (-140.3723, -37.5451) ccw
  arc A121 (-143.0876, -17.6947) -> (-141.7354, -19.6252) centre (-141.4462, -17.9838) ccw
  arc A122 (-138.2556, 0.1266) -> (-140.1864, -1.2256) centre (-138.545, -1.5147) ccw
  arc A123 (-164.5843, -2.8728) -> (-166.5156, -1.521) centre (-166.2256, -3.1623) ccw
  arc A124 (-156.4098, -20.7686) -> (-158.3407, -19.4167) centre (-158.0512, -21.058) ccw
  arc A125 (-154.8721, -39.098) -> (-153.5181, -37.1669) centre (-155.1595, -37.4563) ccw
  arc A126 (-154.4961, -59.04) -> (-156.4246, -57.6876) centre (-156.1374, -59.3294) ccw
  arc A127 (-152.9422, -77.4605) -> (-151.5886, -75.5295) centre (-153.23, -75.8189) ccw
  arc A128 (-159.0128, -97.9408) -> (-157.6604, -96.0106) centre (-159.3018, -96.2994) ccw
  arc A129 (-233.2721, -110.9177) -> (-232.6973, -110.9171) centre (-232.9864, -109.2757) ccw
  arc A130 (-238.1216, -110.0736) -> (-238.407, -110.049) centre (-238.4074, -111.7156) ccw
  arc A131 (-314.919, -108.3659) -> (-313.2527, -110.0326) centre (-313.2523, -108.3659) ccw
  arc A132 (-319.6815, -89.3845) -> (-318.0141, -91.0512) centre (-318.0148, -89.3845) ccw
  arc A133 (-321.5862, -70.3377) -> (-319.919, -72.0043) centre (-319.9196, -70.3377) ccw
  arc A134 (-319.9205, -51.9603) -> (-321.5862, -53.627) centre (-319.9196, -53.627) ccw
  arc A135 (-303.7283, -32.928) -> (-305.3937, -34.5947) centre (-303.7271, -34.5947) ccw
  arc A136 (-284.6776, -13.7995) -> (-286.3442, -15.4662) centre (-284.6776, -15.4662) ccw
  arc A137 (-290.104, -10.7013) -> (-291.7706, -9.0321) centre (-291.7707, -10.6987) ccw
  arc A138 (-237.7191, -15.4662) -> (-239.3858, -13.7995) centre (-239.3858, -15.4662) ccw
  arc A139 (-237.7191, -31.0628) -> (-235.9174, -32.724) centre (-236.0525, -31.0628) ccw
  arc A140 (-229.6794, -31.998) -> (-228.2881, -30.061) centre (-229.9295, -30.3502) ccw
  arc A141 (-229.6592, -12.6764) -> (-231.0106, -14.6069) centre (-229.3692, -14.3177) ccw
  arc A142 (-291.7971, -29.0488) -> (-290.1298, -27.3847) centre (-291.7965, -27.3821) ccw
  arc A143 (-310.7973, -48.0603) -> (-309.1294, -46.3914) centre (-310.796, -46.3936) ccw
  arc A144 (-329.2843, -46.3744) -> (-327.619, -48.0472) centre (-327.6177, -46.3805) ccw
  arc A145 (-348.2579, -27.4277) -> (-346.5912, -29.0945) centre (-346.5913, -27.4278) ccw
  arc A146 (-346.5901, -9.0287) -> (-348.2569, -10.6952) centre (-346.5902, -10.6953) ccw
  dimension "d39" = 19.05
  dimension "d41" = 19.05
  dimension "d47" = 8.5
  dimension "d51" = 8.25
  dimension "d52" = 8.25
  dimension "d53" = 8.25
  dimension "d129" = 1.6667
  dimension "d130" = 1.6667
  constraint parallel L173 L378
  constraint parallel L10 L377
  constraint parallel L202 L376
  constraint parallel L19 L369
  constraint parallel L261 L358
  constraint parallel L191 L359
  constraint parallel L183 L360
  constraint parallel L21 L361
  constraint parallel L3 L362
  constraint parallel L33 L368
  constraint perpendicular L367 L381
  constraint perpendicular L369 L386
  constraint perpendicular L370 L387
  constraint parallel L382 L396
  constraint perpendicular L382 L397
  constraint perpendicular L362 L400
  constraint coincident A71.end L338.start
  constraint coincident L315.end A49.start
  constraint coincident A50.end L317.start
  constraint coincident L321.end A55.end
  constraint coincident L322.end A56.end
  constraint coincident L326.end A60.start
  constraint coincident A60.end L327.start
  constraint coincident A64.start L331.start
  constraint coincident A65.start L332.start
  constraint coincident L336.end A70.start
  constraint coincident L311.start L314.end
  constraint coincident L312.end L313.start
  constraint coincident L311.end L312.start
  constraint coincident L313.end L314.start
  constraint coincident L193.end L194.start
  constraint coincident L192.start L195.end
  constraint coincident L192.end L193.start
  constraint coincident L194.end L195.start
  constraint coincident L30.end L31.start
  constraint coincident L28.end L29.start
  constraint coincident L29.end L30.start
  constraint coincident L28.start L31.end
  constraint midpoint L429 A101.centre
  constraint midpoint L428 A102.centre
  constraint midpoint L426 A103.centre
  constraint perpendicular L372 L391
  constraint concentric A87 A105
  constraint parallel L405 L470
  constraint parallel L394 L471
  constraint parallel L395 L472
  constraint parallel L393 L473
  constraint parallel L371 L474
  constraint parallel L392 L475
  constraint parallel L372 L476
  constraint parallel L391 L477
  constraint parallel L354 L478
  constraint parallel L431 L479
  constraint parallel L433 L480
  constraint parallel L432 L481
  constraint parallel L356 L482
  constraint parallel L390 L483
  constraint parallel L373 L484
  constraint parallel L389 L485
  constraint parallel L374 L486
  constraint parallel L388 L487
  constraint parallel L375 L488
  constraint parallel L387 L489
  constraint parallel L370 L490
  constraint parallel L396 L491
  constraint parallel L397 L492
  constraint tangent L470 A106
  constraint tangent L471 A106
  constraint tangent A105 A107
  constraint tangent L470 A107
  constraint equal A106 A107
  constraint tangent A105 A108
  constraint tangent L492 A108
  constraint equal A106 A108
  constraint tangent L491 A109
  constraint tangent L492 A109
  constraint equal A106 A109
  constraint tangent L471 A110
  constraint tangent L472 A110
  constraint equal A106 A110
  constraint tangent L472 A111
  constraint tangent L473 A111
  constraint equal A106 A111
  constraint tangent L474 A112
  constraint tangent L475 A112
  constraint equal A106 A112
  constraint tangent L476 A113
  constraint tangent L477 A113
  constraint equal A106 A113
  constraint tangent L478 A114
  constraint tangent L479 A114
  constraint equal A106 A114
  constraint tangent L479 A115
  constraint tangent L480 A115
  constraint equal A106 A115
  constraint tangent L480 A116
  constraint tangent L481 A116
  constraint equal A106 A116
  constraint tangent L481 A117
  constraint tangent L482 A117
  constraint equal A106 A117
  constraint tangent L482 A118
  constraint tangent L483 A118
  constraint equal A106 A118
  constraint tangent L485 A119
  constraint tangent L486 A119
  constraint equal A106 A119
  constraint tangent L487 A120
  constraint tangent L488 A120
  constraint equal A106 A120
  constraint tangent L489 A121
  constraint tangent L490 A121
  constraint equal A106 A121
  constraint tangent L490 A122
  constraint tangent L491 A122
  constraint equal A106 A122
  constraint parallel L358 L437
  constraint parallel L404 L438
  constraint parallel L359 L439
  constraint parallel L403 L440
  constraint parallel L360 L441
  constraint parallel L402 L442
  constraint parallel L361 L443
  constraint parallel L401 L444
  constraint parallel L362 L445
  constraint parallel L400 L446
  constraint parallel L368 L447
  constraint concentric A88 A104
  constraint parallel L399 L448
  constraint parallel L398 L449
  constraint parallel L369 L450
  constraint parallel L386 L451
  constraint parallel L376 L452
  constraint parallel L385 L453
  constraint parallel L377 L454
  constraint parallel L384 L455
  constraint parallel L378 L456
  constraint parallel L383 L457
  constraint parallel L357 L458
  constraint parallel L434 L459
  constraint parallel L435 L460
  constraint parallel L436 L461
  constraint tangent L449 A123
  constraint tangent L450 A123
  constraint equal A106 A123
  constraint tangent L451 A124
  constraint tangent L452 A124
  constraint equal A106 A124
  constraint tangent L452 A125
  constraint tangent L453 A125
  constraint equal A106 A125
  constraint tangent L455 A126
  constraint tangent L456 A126
  constraint equal A106 A126
  constraint tangent L456 A127
  constraint tangent L457 A127
  constraint tangent L458 A128
  constraint tangent L459 A128
  constraint equal A127 A128
  constraint tangent L459 A129
  constraint tangent L460 A129
  constraint equal A127 A129
  constraint tangent L460 A130
  constraint tangent L461 A130
  constraint equal A127 A130
  constraint tangent L437 A131
  constraint tangent L461 A131
  constraint equal A127 A131
  constraint tangent L438 A132
  constraint tangent L439 A132
  constraint equal A127 A132
  constraint tangent L440 A133
  constraint tangent L441 A133
  constraint equal A127 A133
  constraint tangent L441 A134
  constraint tangent L442 A134
  constraint equal A127 A134
  constraint tangent L443 A135
  constraint tangent L444 A135
  constraint equal A127 A135
  constraint tangent L445 A136
  constraint tangent L446 A136
  constraint equal A127 A136
  constraint parallel L367 L462
  constraint parallel L381 L463
  constraint parallel L366 L464
  constraint parallel L379 L465
  constraint parallel L363 L466
  constraint parallel L364 L467
  constraint parallel L365 L468
  constraint parallel L380 L469
  constraint tangent L463 A137
  constraint tangent L464 A137
  constraint equal A127 A137
  constraint tangent L446 A138
  constraint tangent L447 A138
  constraint equal A127 A138
  constraint tangent L447 A139
  constraint tangent A104 A139
  constraint equal A127 A139
  constraint tangent A104 A140
  constraint tangent L448 A140
  constraint equal A127 A140
  constraint tangent L448 A141
  constraint tangent L449 A141
  constraint equal A127 A141
  constraint tangent L464 A142
  constraint tangent L465 A142
  constraint equal A127 A142
  constraint tangent L466 A143
  constraint tangent L467 A143
  constraint equal A127 A143
  constraint tangent L467 A144
  constraint tangent L468 A144
  constraint equal A127 A144
  constraint tangent L462 A145
  constraint tangent L469 A145
  constraint equal A127 A145
  constraint tangent L462 A146
  constraint tangent L463 A146
  constraint equal A127 A146
  measures "d39" distance of L396.start L382.end
  measures "d41" distance of L398.end L399.end
  measures "d51" diameter of A101
  measures "d52" diameter of A102
  measures "d53" diameter of A103
  measures "d129" radius of A106
  measures "d130" radius of A127
extrude "top profile (1)" add sketch "top profile" along normal blind 5 separate body contours A0 | L28 L29 L30 L31 | A1 | L192 L193 L194 L195 | A34 | A39 | A40 | A45 | A46 | A47 | L311 L312 L313 L314 | L315 A49 L316 A50 L317 L321 A55 L322 L326 A60 L327 L331 A65 L332 L336 A70 L337 A71 L338 L342 L346 L350 L407 A89 A90 A91 A92 A93 L408 L409 A94 L410 A95 L411 L412 L413 L414 L415 | A48 A84 L351 A85 L352 A86 L353 L411 | A80 L347 A81 L348 A82 L349 A83 L411 | A76 L343 A77 L344 A78 L345 A79 L411 | A51 L318 A52 L319 A53 L320 A54 L412 | A72 L339 A73 L340 A74 L341 A75 L411 | A56 L323 A57 L324 A58 L325 A59 L413 | A66 L333 A67 L334 A68 L335 A69 L415 | A61 L328 A62 L329 A63 L330 A64 L414 | L416 A96 L417 A97 L418 L419 L420 A98 L421 L422 L423 A99 L424 A100 makes body 2
extrude "bottom of the top" add 1 faces at (360.3629, 60.5187, 1.6) along direction (0, 0, -1) blind 7 on bodies 2 bodies 2